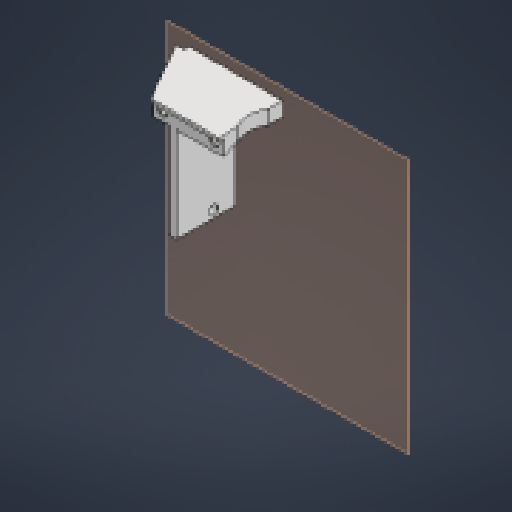
# Autodesk Inventor part: bok
Saved by Autodesk Inventor 2023 (Build 270158000, 158)
## iProperties
Created: 2024-02-25
Part Number: bok
Material: Generic
Document SubType Name: Modeling
Designer: Michał
Density: 1 g/cm^3
Appearance: Default
Author: Michał
Autodesk Inventor part; units mm, degrees
ref_plane "YZ Plane" through (0, 0, 0) normal (1, 0, 0) x (0, 1, 0)
ref_plane "XZ Plane" through (0, 0, 0) normal (0, 1, 0) x (-1, 0, 0)
ref_plane "XY Plane" through (0, 0, 0) normal (0, 0, 1) x (1, 0, 0)
ref_plane "Work Plane1" through (0, 0, 0) normal (0, 0, 1) x (1, 0, 0)
sketch "Sketch1" plane through (0, 0, 0) normal (0, 0, 1) x (1, 0, 0)
  line L0 (22.75, 48.75) -> (-33.25, 48.75) construction
  line L1 (-46.45, 48.75) -> (-46.45, 42.75)
  line L2 (-21.95, 42.75) -> (-26.45, 42.75)
  line L3 (-26.45, 42.75) -> (-26.45, 0.75)
  line L4 (-26.45, 0.75) -> (-21.95, 0.75)
  line L5 (-21.95, 0.75) -> (-21.95, 42.75)
  line L6 (-46.45, 49) -> (-46.45, 41.0784) construction
  line L7 (-46.45, 42.75) -> (-2.25, 42.75)
  line L8 (-2.25, 42.75) -> (-2.25, 48.75)
  line L9 (-2.25, 48.75) -> (-46.45, 48.75)
  line L10 (22.75, -48.75) -> (22.75, 48.75) construction
  point P0 (0, 0)
  dimension "d1" = 20
  dimension "d2" = 4.5
  dimension "d23" = 25
  dimension "d24" = 6
  dimension "d25" = 48
  constraints: 16 end point, 3 horizontal, 2 collinear, 2 parallel, 2 perpendicular, 1 point on line
  measures "d1" distance between parallel lines of L3 L1
  measures "d2" distance between parallel lines of L5 L3
  measures "d23" distance between parallel lines of L10 L8
  measures "d24" distance between parallel lines of L9 L7
  measures "d25" distance from line of L9 L3.end
extrude "Extrusion1" add sketch "Sketch1" along normal blind 25
chamfer "Chamfer2" distance 25 angle 3.5 1 edges at (-26.45, 21.75, 25) measured on face at (-26.45, 28.75, 8.3333)
sketch "Sketch2" plane through (-26.45, 0.75, 0) normal (-0.9981348, 0, 0.0610485) x (0.0610485, 0, 0.9981348)
  line L0 (0, 0) -> (25.0467, 0) construction
  line L1 (0, 42) -> (0, 0) construction
  line L2 (9.75, 39) -> (9.75, 3) construction
  point P0 (1.6147, -0.75)
  point P1 (9.75, 21)
  point P2 (0, 21)
  dimension "d12" = 36
  dimension "d13" = 9.75
  constraints: 2 end point, 2 midpoint, 1 horizontal alignment, 1 vertical, 1 vertical alignment
  measures "d12" distance of L2.end L2.start
  measures "d13" distance from line of L2.end L1
hole "Hole1" at (-25.8548, 39.75, 9.7318) at (-25.8548, 3.75, 9.7318) direction (0.9981348, 0, -0.0610485) diameter 4 depth 4 counterbore diameter 4.5 counterbore depth 0.6
sketch "Sketch4" plane through (-2.25, 48.75, 25) normal (0, 1, 0) x (1, 0, 0)
  circle A0 centre (10.5, 12.5) radius 12.2 construction
  circle A1 centre (10.5, 12.5) radius 12.4
  dimension "d42" = 0.2
  constraints: 1 centre point
  measures "d42" radial gap between concentric circles of A1 A0
extrude "Extrusion3" cut sketch "Sketch4" against normal through all
sketch "Sketch5" plane through (0, 0, 25) normal (0, 0, 1) x (1, 0, 0)
  line L0 (-46.45, 48.75) -> (-46.45, 42.75) projected
  line L1 (-2.25, 48.75) -> (-46.45, 48.75)
  line L2 (-46.45, 48.75) -> (-46.45, 47.25)
  line L3 (-46.45, 47.25) -> (-2.25, 47.25)
  line L4 (-2.25, 47.25) -> (-2.25, 48.75)
  point P0 (0, 0)
  dimension "d29" = 1.5
  constraints: 8 end point, 2 parallel, 1 horizontal, 1 perpendicular, 1 point on line
  measures "d29" distance between parallel lines of L3 L1
extrude "Extrusion4" add sketch "Sketch5" along normal blind 2
sketch "Sketch3" plane through (22.75, 48.75, 25) normal (0, 1, 0) x (1, 0, 0)
  line L0 (-69.2, 23) -> (-64.5, 23) projected
  line L1 (-64.5, 23) -> (-64.5, 25) projected
  line L2 (-64.5, 25) -> (-69, 25) projected
  line L3 (-69, 25) -> (-69, 27.5) projected
  line L4 (-69, 27.5) -> (-73.7, 27.5) projected
  line L5 (-73.7, 27.5) -> (-69.2, 23) projected
  line L6 (-64.3, 22.8) -> (-69.2828, 22.8)
  line L7 (-69.2828, 22.8) -> (-74.1828, 27.7)
  line L8 (-74.1828, 27.7) -> (-68.8, 27.7)
  line L9 (-68.8, 27.7) -> (-68.8, 25.2)
  line L10 (-68.8, 25.2) -> (-64.3, 25.2)
  line L11 (-64.3, 25.2) -> (-64.3, 22.8)
  line L12 (-69.2, 25) -> (-69.2, -2) projected
  line L13 (-69.2, 22.8) -> (-54.8817, -2)
  line L14 (-54.8817, -2) -> (-69.2, -2)
  line L15 (-69.2, -2) -> (-69.2, 22.8)
  line L16 (-54.8817, -2) -> (-53.4961, -2)
  line L17 (-25, -2) -> (-69.2, -2) projected
  line L18 (-67.8144, 22.8) -> (-53.4961, -2)
  point P0 (-22.75, 25)
  point P1 (-68.85, 25.15)
  point P2 (-68.7, 25)
  dimension "d32" = 0.2
  dimension "d33" = 30
  dimension "d34" = 1.2
  constraints: 22 end point, 4 point on line, 1 horizontal, 1 parallel, 5 other
  measures "d32" distance between parallel lines of L6 L0
  measures "d33" angle of L12 L13
  measures "d34" distance between parallel lines of L13 L18
extrude "Extrusion2" cut sketch "Sketch3" against normal through all contours L5 L4 L3 L2 L1 L0 | L6 L7 L8 L9 L10 L11 | L18 L16 L13 L6 | L13 L14 L12
sketch "Sketch6" plane through (0, 0, 0) normal (0, 0, -1) x (-1, 0, 0)
  arc A0 (7.2895, 48.75) -> (9.2105, 48.75) centre (8.25, 45.75) ccw construction
  arc A1 (29.2895, 48.75) -> (33.25, 44.7895) centre (30.25, 45.75) ccw construction
  point P0 (0, 0)
  constraints: 2 coincident
hole "Hole2" at (-8.25, 45.75, 0) at (-30.25, 45.75, 0) direction (0, 0, 1) diameter 4 depth 4 counterbore diameter 4.5 counterbore depth 0.6
sketch "Sketch7" plane through (0, 0, 25) normal (0, 0, 1) x (1, 0, 0)
  line L0 (-2.25, 42.75) -> (-2.25, 47.25) construction
  line L1 (-31.9008, 47.25) -> (-31.9008, 42.75) construction
  point P0 (0, 0)
  point P1 (-6.25, 45)
  point P2 (-27.9008, 45)
  point P3 (-2.25, 45)
  point P4 (-2.25, 45)
  dimension "d43" = 4
  dimension "d44" = 4
  constraints: 2 horizontal alignment, 2 midpoint
  measures "d43" distance of point (-2.25, 45) point (-6.25, 45)
  measures "d44" distance from line of L1 point (-27.901, 45)
hole "Hole3" at (-27.9008, 45, 25) at (-6.25, 45, 25) direction (0, 0, -1) diameter 4 depth 4 counterbore diameter 4.5 counterbore depth 0.6
sketch "Sketch8" plane through (-2.25, 42.75, 19.0962) normal (1, 0, 0) x (0, 0, -1)
  line L0 (-5.9038, 0) -> (19.0962, 0) projected
  line L1 (-1.4038, 0) -> (-5.9038, -2)
  line L2 (-5.9038, -42) -> (-5.9038, 0) projected
  line L3 (-5.9038, 0) -> (-5.9038, -2)
  point P0 (19.0962, -42.75)
  dimension "d52" = 4.5
  dimension "d53" = 2
  constraints: 4 end point, 2 point on line, 1 collinear
  measures "d52" distance from line of L2 L1.start
  measures "d53" distance from line of L0 L1.end
extrude "Extrusion5" add sketch "Sketch8" against normal up to surface surface through (-45.0644, 48.75, 2.2) normal (0.8660254, 0, -0.5)
body "Solid1"
